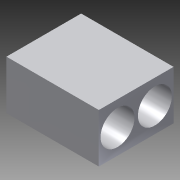
# Autodesk Inventor part: TE_2Pin
Saved by Autodesk Inventor 2014 (Build 180170000, 170)
## iProperties
Created: 2015-04-19
Part Number: TE_2Pin
Material: Generic
Document SubType Name: Modeling
Designer: Owner
Density: 1 g/cm^3
Appearance: White
Author: Owner
Autodesk Inventor part; units mm, degrees
ref_plane "YZ Plane" through (0, 0, 0) normal (1, 0, 0) x (0, 1, 0)
ref_plane "XZ Plane" through (0, 0, 0) normal (0, 1, 0) x (-1, 0, 0)
ref_plane "XY Plane" through (0, 0, 0) normal (0, 0, 1) x (1, 0, 0)
sketch "Sketch1" plane through (0, 0, 0) normal (0, 1, 0) x (-1, 0, 0)
  line L0 (-10.8149, 6.985) -> (6.4571, 6.985)
  line L1 (6.4571, 6.985) -> (6.4571, -6.985)
  line L2 (6.4571, -6.985) -> (-10.8149, -6.985)
  line L3 (-10.8149, -6.985) -> (-10.8149, 6.985)
  point P0 (0, 0)
  dimension "d0" = 13.97
  dimension "d1" = 17.272
  dimension "d2" = 6.985
  constraints: 8 end point, 2 parallel, 1 horizontal, 1 perpendicular
  measures "d0" distance of L0.end L1.end
  measures "d1" distance of L0.start L0.end
  measures "d2" distance from line of L0 point (0, 0)
extrude "Extrusion1" add sketch "Sketch1" along normal blind 9.144
sketch "Sketch3" plane through (10.8149, 0, 6.985) normal (1, 0, 0) x (0, 0, -1)
  line L0 (13.97, 0) -> (13.97, 9.144) projected
  line L1 (0, 0) -> (0, 9.144) projected
  circle A0 centre (3.4925, 4.572) radius 3.175
  circle A1 centre (10.4775, 4.572) radius 3.175
  point P0 (6.985, 0)
  dimension "d6" = 6.35
  dimension "d7" = 6.35
  dimension "d8" = 3.4925
  dimension "d9" = 3.4925
  constraints: 2 centre point
  measures "d6" diameter of A0
  measures "d7" diameter of A1
  measures "d8" distance from line of L1 A0.centre
  measures "d9" distance from line of L0 A1.centre
extrude "Extrusion2" cut sketch "Sketch3" against normal blind 4.572
body "Solid1"
